Autodesk Inventor part; units mm, degrees
(part 2 of 2)
sketch "Sketch5" plane through (0, 0, 0) normal (0, -1, 0) x (1, 0, 0)
  circle A0 centre (-0.4117, 0.4117) radius 0.057 projected
  line L0 (-0.0797, 0.4378) -> (-0.0785, 0.4393) projected
  line L1 (-0.0785, 0.4393) -> (-0.0772, 0.4404) projected
  line L2 (-0.0772, 0.4404) -> (-0.076, 0.4413) projected
  line L3 (-0.076, 0.4413) -> (-0.0747, 0.442) projected
  line L4 (-0.0747, 0.442) -> (-0.0734, 0.4426) projected
  line L5 (-0.0734, 0.4426) -> (-0.0708, 0.4437) projected
  line L6 (-0.0708, 0.4437) -> (-0.0682, 0.4445) projected
  line L7 (-0.0682, 0.4445) -> (-0.0656, 0.4451) projected
  line L8 (-0.0656, 0.4451) -> (-0.0604, 0.4462) projected
  line L9 (-0.0604, 0.4462) -> (-0.0552, 0.4478) projected
  line L10 (-0.0552, 0.4478) -> (-0.05, 0.4497) projected
  line L11 (-0.05, 0.4497) -> (-0.0449, 0.452) projected
  line L12 (-0.0449, 0.452) -> (-0.0398, 0.4545) projected
  line L13 (-0.0398, 0.4545) -> (-0.0348, 0.4573) projected
  line L14 (-0.0348, 0.4573) -> (-0.0298, 0.4603) projected
  line L15 (-0.0298, 0.4603) -> (-0.0248, 0.4636) projected
  line L16 (-0.0248, 0.4636) -> (-0.0199, 0.467) projected
  line L17 (-0.0199, 0.467) -> (-0.015, 0.4707) projected
  line L18 (-0.015, 0.4707) -> (-0.0102, 0.4745) projected
  line L19 (-0.0102, 0.4745) -> (-0.0055, 0.4786) projected
  line L20 (-0.0055, 0.4786) -> (-0.0167, 0.5276) projected
  line L21 (-0.0167, 0.5276) -> (-0.0227, 0.5292) projected
  line L22 (-0.0227, 0.5292) -> (-0.0287, 0.5306) projected
  line L23 (-0.0287, 0.5306) -> (-0.0347, 0.5318) projected
  line L24 (-0.0347, 0.5318) -> (-0.0406, 0.5328) projected
  line L25 (-0.0406, 0.5328) -> (-0.0465, 0.5335) projected
  line L26 (-0.0465, 0.5335) -> (-0.0523, 0.5341) projected
  line L27 (-0.0523, 0.5341) -> (-0.058, 0.5344) projected
  line L28 (-0.058, 0.5344) -> (-0.0637, 0.5345) projected
  line L29 (-0.0637, 0.5345) -> (-0.0693, 0.5343) projected
  line L30 (-0.0693, 0.5343) -> (-0.0748, 0.5338) projected
  line L31 (-0.0748, 0.5338) -> (-0.0802, 0.5329) projected
  line L32 (-0.0802, 0.5329) -> (-0.0854, 0.5316) projected
  line L33 (-0.0854, 0.5316) -> (-0.088, 0.5311) projected
  line L34 (-0.088, 0.5311) -> (-0.0907, 0.5307) projected
  line L35 (-0.0907, 0.5307) -> (-0.0935, 0.5305) projected
  line L36 (-0.0935, 0.5305) -> (-0.0949, 0.5305) projected
  line L37 (-0.0949, 0.5305) -> (-0.0964, 0.5307) projected
  line L38 (-0.0964, 0.5307) -> (-0.0979, 0.5309) projected
  line L39 (-0.0979, 0.5309) -> (-0.0995, 0.5313) projected
  line L40 (-0.0995, 0.5313) -> (-0.1012, 0.5322) projected
  line L41 (-0.1012, 0.5322) -> (-0.1038, 0.535) projected
  line L42 (-0.1038, 0.535) -> (-0.1233, 0.5755) projected
  line L43 (-0.1233, 0.5755) -> (-0.1239, 0.5792) projected
  line L44 (-0.1239, 0.5792) -> (-0.1235, 0.5811) projected
  line L45 (-0.1235, 0.5811) -> (-0.1228, 0.5826) projected
  line L46 (-0.1228, 0.5826) -> (-0.1221, 0.584) projected
  line L47 (-0.1221, 0.584) -> (-0.1212, 0.5852) projected
  line L48 (-0.1212, 0.5852) -> (-0.1204, 0.5863) projected
  line L49 (-0.1204, 0.5863) -> (-0.1185, 0.5884) projected
  line L50 (-0.1185, 0.5884) -> (-0.1165, 0.5903) projected
  line L51 (-0.1165, 0.5903) -> (-0.1144, 0.592) projected
  line L52 (-0.1144, 0.592) -> (-0.1102, 0.5952) projected
  line L53 (-0.1102, 0.5952) -> (-0.1061, 0.5989) projected
  line L54 (-0.1061, 0.5989) -> (-0.1023, 0.6029) projected
  line L55 (-0.1023, 0.6029) -> (-0.0987, 0.6071) projected
  line L56 (-0.0987, 0.6071) -> (-0.0952, 0.6116) projected
  line L57 (-0.0952, 0.6116) -> (-0.0919, 0.6163) projected
  line L58 (-0.0919, 0.6163) -> (-0.0887, 0.6212) projected
  line L59 (-0.0887, 0.6212) -> (-0.0856, 0.6263) projected
  line L60 (-0.0856, 0.6263) -> (-0.0827, 0.6315) projected
  line L61 (-0.0827, 0.6315) -> (-0.0799, 0.6369) projected
  line L62 (-0.0799, 0.6369) -> (-0.0773, 0.6425) projected
  line L63 (-0.0773, 0.6425) -> (-0.0747, 0.6482) projected
  line L64 (-0.0747, 0.6482) -> (-0.1061, 0.6875) projected
  line L65 (-0.1061, 0.6875) -> (-0.1122, 0.6863) projected
  line L66 (-0.1122, 0.6863) -> (-0.1182, 0.685) projected
  line L67 (-0.1182, 0.685) -> (-0.1241, 0.6835) projected
  line L68 (-0.1241, 0.6835) -> (-0.1299, 0.6818) projected
  line L69 (-0.1299, 0.6818) -> (-0.1355, 0.6799) projected
  line L70 (-0.1355, 0.6799) -> (-0.141, 0.6779) projected
  line L71 (-0.141, 0.6779) -> (-0.1463, 0.6757) projected
  line L72 (-0.1463, 0.6757) -> (-0.1515, 0.6733) projected
  line L73 (-0.1515, 0.6733) -> (-0.1564, 0.6707) projected
  line L74 (-0.1564, 0.6707) -> (-0.1612, 0.6679) projected
  line L75 (-0.1612, 0.6679) -> (-0.1656, 0.6648) projected
  line L76 (-0.1656, 0.6648) -> (-0.1697, 0.6613) projected
  line L77 (-0.1697, 0.6613) -> (-0.1719, 0.6597) projected
  line L78 (-0.1719, 0.6597) -> (-0.1741, 0.6582) projected
  line L79 (-0.1741, 0.6582) -> (-0.1766, 0.6568) projected
  line L80 (-0.1766, 0.6568) -> (-0.1779, 0.6562) projected
  line L81 (-0.1779, 0.6562) -> (-0.1792, 0.6557) projected
  line L82 (-0.1792, 0.6557) -> (-0.1807, 0.6552) projected
  line L83 (-0.1807, 0.6552) -> (-0.1823, 0.6549) projected
  line L84 (-0.1823, 0.6549) -> (-0.1843, 0.6549) projected
  line L85 (-0.1843, 0.6549) -> (-0.1878, 0.6564) projected
  line L86 (-0.1878, 0.6564) -> (-0.2229, 0.6844) projected
  line L87 (-0.2229, 0.6844) -> (-0.2251, 0.6875) projected
  line L88 (-0.2251, 0.6875) -> (-0.2255, 0.6894) projected
  line L89 (-0.2255, 0.6894) -> (-0.2256, 0.691) projected
  line L90 (-0.2256, 0.691) -> (-0.2255, 0.6926) projected
  line L91 (-0.2255, 0.6926) -> (-0.2253, 0.694) projected
  line L92 (-0.2253, 0.694) -> (-0.225, 0.6954) projected
  line L93 (-0.225, 0.6954) -> (-0.2242, 0.6981) projected
  line L94 (-0.2242, 0.6981) -> (-0.2232, 0.7006) projected
  line L95 (-0.2232, 0.7006) -> (-0.2221, 0.7031) projected
  line L96 (-0.2221, 0.7031) -> (-0.2197, 0.7079) projected
  line L97 (-0.2197, 0.7079) -> (-0.2176, 0.7129) projected
  line L98 (-0.2176, 0.7129) -> (-0.2159, 0.7181) projected
  line L99 (-0.2159, 0.7181) -> (-0.2145, 0.7236) projected
  line L100 (-0.2145, 0.7236) -> (-0.2133, 0.7291) projected
  line L101 (-0.2133, 0.7291) -> (-0.2123, 0.7348) projected
  line L102 (-0.2123, 0.7348) -> (-0.2116, 0.7406) projected
  line L103 (-0.2116, 0.7406) -> (-0.211, 0.7465) projected
  line L104 (-0.211, 0.7465) -> (-0.2107, 0.7525) projected
  line L105 (-0.2107, 0.7525) -> (-0.2105, 0.7585) projected
  line L106 (-0.2105, 0.7585) -> (-0.2105, 0.7647) projected
  line L107 (-0.2105, 0.7647) -> (-0.2107, 0.771) projected
  line L108 (-0.2107, 0.771) -> (-0.256, 0.7928) projected
  line L109 (-0.256, 0.7928) -> (-0.261, 0.789) projected
  line L110 (-0.261, 0.789) -> (-0.2659, 0.7852) projected
  line L111 (-0.2659, 0.7852) -> (-0.2705, 0.7813) projected
  line L112 (-0.2705, 0.7813) -> (-0.275, 0.7773) projected
  line L113 (-0.275, 0.7773) -> (-0.2793, 0.7732) projected
  line L114 (-0.2793, 0.7732) -> (-0.2833, 0.769) projected
  line L115 (-0.2833, 0.769) -> (-0.2872, 0.7647) projected
  line L116 (-0.2872, 0.7647) -> (-0.2908, 0.7603) projected
  line L117 (-0.2908, 0.7603) -> (-0.2941, 0.7558) projected
  line L118 (-0.2941, 0.7558) -> (-0.2971, 0.7512) projected
  line L119 (-0.2971, 0.7512) -> (-0.2998, 0.7465) projected
  line L120 (-0.2998, 0.7465) -> (-0.302, 0.7416) projected
  line L121 (-0.302, 0.7416) -> (-0.3032, 0.7392) projected
  line L122 (-0.3032, 0.7392) -> (-0.3046, 0.7368) projected
  line L123 (-0.3046, 0.7368) -> (-0.3062, 0.7345) projected
  line L124 (-0.3062, 0.7345) -> (-0.3071, 0.7334) projected
  line L125 (-0.3071, 0.7334) -> (-0.3081, 0.7323) projected
  line L126 (-0.3081, 0.7323) -> (-0.3093, 0.7313) projected
  line L127 (-0.3093, 0.7313) -> (-0.3106, 0.7303) projected
  line L128 (-0.3106, 0.7303) -> (-0.3123, 0.7295) projected
  line L129 (-0.3123, 0.7295) -> (-0.3161, 0.7293) projected
  line L130 (-0.3161, 0.7293) -> (-0.3599, 0.7393) projected
  line L131 (-0.3599, 0.7393) -> (-0.3633, 0.7411) projected
  line L132 (-0.3633, 0.7411) -> (-0.3644, 0.7426) projected
  line L133 (-0.3644, 0.7426) -> (-0.3652, 0.7441) projected
  line L134 (-0.3652, 0.7441) -> (-0.3658, 0.7455) projected
  line L135 (-0.3658, 0.7455) -> (-0.3663, 0.7469) projected
  line L136 (-0.3663, 0.7469) -> (-0.3666, 0.7483) projected
  line L137 (-0.3666, 0.7483) -> (-0.3671, 0.7511) projected
  line L138 (-0.3671, 0.7511) -> (-0.3673, 0.7538) projected
  line L139 (-0.3673, 0.7538) -> (-0.3673, 0.7565) projected
  line L140 (-0.3673, 0.7565) -> (-0.3672, 0.7618) projected
  line L141 (-0.3672, 0.7618) -> (-0.3676, 0.7673) projected
  line L142 (-0.3676, 0.7673) -> (-0.3683, 0.7727) projected
  line L143 (-0.3683, 0.7727) -> (-0.3694, 0.7782) projected
  line L144 (-0.3694, 0.7782) -> (-0.3707, 0.7837) projected
  line L145 (-0.3707, 0.7837) -> (-0.3723, 0.7893) projected
  line L146 (-0.3723, 0.7893) -> (-0.3741, 0.7948) projected
  line L147 (-0.3741, 0.7948) -> (-0.3762, 0.8004) projected
  line L148 (-0.3762, 0.8004) -> (-0.3784, 0.8059) projected
  line L149 (-0.3784, 0.8059) -> (-0.3809, 0.8115) projected
  line L150 (-0.3809, 0.8115) -> (-0.3836, 0.817) projected
  line L151 (-0.3836, 0.817) -> (-0.3865, 0.8226) projected
  line L152 (-0.3865, 0.8226) -> (-0.4368, 0.8226) projected
  line L153 (-0.4368, 0.8226) -> (-0.4397, 0.817) projected
  line L154 (-0.4397, 0.817) -> (-0.4424, 0.8115) projected
  line L155 (-0.4424, 0.8115) -> (-0.4449, 0.8059) projected
  line L156 (-0.4449, 0.8059) -> (-0.4472, 0.8004) projected
  line L157 (-0.4472, 0.8004) -> (-0.4492, 0.7948) projected
  line L158 (-0.4492, 0.7948) -> (-0.4511, 0.7893) projected
  line L159 (-0.4511, 0.7893) -> (-0.4527, 0.7837) projected
  line L160 (-0.4527, 0.7837) -> (-0.454, 0.7782) projected
  line L161 (-0.454, 0.7782) -> (-0.455, 0.7727) projected
  line L162 (-0.455, 0.7727) -> (-0.4558, 0.7673) projected
  line L163 (-0.4558, 0.7673) -> (-0.4561, 0.7618) projected
  line L164 (-0.4561, 0.7618) -> (-0.456, 0.7565) projected
  line L165 (-0.456, 0.7565) -> (-0.4561, 0.7538) projected
  line L166 (-0.4561, 0.7538) -> (-0.4563, 0.7511) projected
  line L167 (-0.4563, 0.7511) -> (-0.4567, 0.7483) projected
  line L168 (-0.4567, 0.7483) -> (-0.4571, 0.7469) projected
  line L169 (-0.4571, 0.7469) -> (-0.4575, 0.7455) projected
  line L170 (-0.4575, 0.7455) -> (-0.4581, 0.7441) projected
  line L171 (-0.4581, 0.7441) -> (-0.4589, 0.7426) projected
  line L172 (-0.4589, 0.7426) -> (-0.4601, 0.7411) projected
  line L173 (-0.4601, 0.7411) -> (-0.4634, 0.7393) projected
  line L174 (-0.4634, 0.7393) -> (-0.5072, 0.7293) projected
  line L175 (-0.5072, 0.7293) -> (-0.511, 0.7295) projected
  line L176 (-0.511, 0.7295) -> (-0.5127, 0.7303) projected
  line L177 (-0.5127, 0.7303) -> (-0.5141, 0.7313) projected
  line L178 (-0.5141, 0.7313) -> (-0.5152, 0.7323) projected
  line L179 (-0.5152, 0.7323) -> (-0.5162, 0.7334) projected
  line L180 (-0.5162, 0.7334) -> (-0.5171, 0.7345) projected
  line L181 (-0.5171, 0.7345) -> (-0.5187, 0.7368) projected
  line L182 (-0.5187, 0.7368) -> (-0.5201, 0.7392) projected
  line L183 (-0.5201, 0.7392) -> (-0.5213, 0.7416) projected
  line L184 (-0.5213, 0.7416) -> (-0.5235, 0.7465) projected
  line L185 (-0.5235, 0.7465) -> (-0.5262, 0.7512) projected
  line L186 (-0.5262, 0.7512) -> (-0.5293, 0.7558) projected
  line L187 (-0.5293, 0.7558) -> (-0.5326, 0.7603) projected
  line L188 (-0.5326, 0.7603) -> (-0.5362, 0.7647) projected
  line L189 (-0.5362, 0.7647) -> (-0.54, 0.769) projected
  line L190 (-0.54, 0.769) -> (-0.5441, 0.7732) projected
  line L191 (-0.5441, 0.7732) -> (-0.5483, 0.7773) projected
  line L192 (-0.5483, 0.7773) -> (-0.5528, 0.7813) projected
  line L193 (-0.5528, 0.7813) -> (-0.5575, 0.7852) projected
  line L194 (-0.5575, 0.7852) -> (-0.5623, 0.789) projected
  line L195 (-0.5623, 0.789) -> (-0.5673, 0.7928) projected
  line L196 (-0.5673, 0.7928) -> (-0.6126, 0.771) projected
  line L197 (-0.6126, 0.771) -> (-0.6128, 0.7647) projected
  line L198 (-0.6128, 0.7647) -> (-0.6128, 0.7585) projected
  line L199 (-0.6128, 0.7585) -> (-0.6127, 0.7525) projected
  line L200 (-0.6127, 0.7525) -> (-0.6123, 0.7465) projected
  line L201 (-0.6123, 0.7465) -> (-0.6118, 0.7406) projected
  line L202 (-0.6118, 0.7406) -> (-0.611, 0.7348) projected
  line L203 (-0.611, 0.7348) -> (-0.61, 0.7291) projected
  line L204 (-0.61, 0.7291) -> (-0.6088, 0.7236) projected
  line L205 (-0.6088, 0.7236) -> (-0.6074, 0.7181) projected
  line L206 (-0.6074, 0.7181) -> (-0.6057, 0.7129) projected
  line L207 (-0.6057, 0.7129) -> (-0.6037, 0.7079) projected
  line L208 (-0.6037, 0.7079) -> (-0.6013, 0.7031) projected
  line L209 (-0.6013, 0.7031) -> (-0.6001, 0.7006) projected
  line L210 (-0.6001, 0.7006) -> (-0.5991, 0.6981) projected
  line L211 (-0.5991, 0.6981) -> (-0.5983, 0.6954) projected
  line L212 (-0.5983, 0.6954) -> (-0.598, 0.694) projected
  line L213 (-0.598, 0.694) -> (-0.5978, 0.6926) projected
  line L214 (-0.5978, 0.6926) -> (-0.5977, 0.691) projected
  line L215 (-0.5977, 0.691) -> (-0.5978, 0.6894) projected
  line L216 (-0.5978, 0.6894) -> (-0.5982, 0.6875) projected
  line L217 (-0.5982, 0.6875) -> (-0.6004, 0.6844) projected
  line L218 (-0.6004, 0.6844) -> (-0.6356, 0.6564) projected
  line L219 (-0.6356, 0.6564) -> (-0.6391, 0.6549) projected
  line L220 (-0.6391, 0.6549) -> (-0.641, 0.6549) projected
  line L221 (-0.641, 0.6549) -> (-0.6426, 0.6552) projected
  line L222 (-0.6426, 0.6552) -> (-0.6441, 0.6557) projected
  line L223 (-0.6441, 0.6557) -> (-0.6455, 0.6562) projected
  line L224 (-0.6455, 0.6562) -> (-0.6468, 0.6568) projected
  line L225 (-0.6468, 0.6568) -> (-0.6492, 0.6582) projected
  line L226 (-0.6492, 0.6582) -> (-0.6515, 0.6597) projected
  line L227 (-0.6515, 0.6597) -> (-0.6536, 0.6613) projected
  line L228 (-0.6536, 0.6613) -> (-0.6577, 0.6648) projected
  line L229 (-0.6577, 0.6648) -> (-0.6622, 0.6679) projected
  line L230 (-0.6622, 0.6679) -> (-0.6669, 0.6707) projected
  line L231 (-0.6669, 0.6707) -> (-0.6719, 0.6733) projected
  line L232 (-0.6719, 0.6733) -> (-0.677, 0.6757) projected
  line L233 (-0.677, 0.6757) -> (-0.6823, 0.6779) projected
  line L234 (-0.6823, 0.6779) -> (-0.6878, 0.6799) projected
  line L235 (-0.6878, 0.6799) -> (-0.6935, 0.6818) projected
  line L236 (-0.6935, 0.6818) -> (-0.6992, 0.6835) projected
  line L237 (-0.6992, 0.6835) -> (-0.7051, 0.685) projected
  line L238 (-0.7051, 0.685) -> (-0.7111, 0.6863) projected
  line L239 (-0.7111, 0.6863) -> (-0.7173, 0.6875) projected
  line L240 (-0.7173, 0.6875) -> (-0.7486, 0.6482) projected
  line L241 (-0.7486, 0.6482) -> (-0.7461, 0.6425) projected
  line L242 (-0.7461, 0.6425) -> (-0.7434, 0.6369) projected
  line L243 (-0.7434, 0.6369) -> (-0.7406, 0.6315) projected
  line L244 (-0.7406, 0.6315) -> (-0.7377, 0.6263) projected
  line L245 (-0.7377, 0.6263) -> (-0.7347, 0.6212) projected
  line L246 (-0.7347, 0.6212) -> (-0.7315, 0.6163) projected
  line L247 (-0.7315, 0.6163) -> (-0.7281, 0.6116) projected
  line L248 (-0.7281, 0.6116) -> (-0.7247, 0.6071) projected
  line L249 (-0.7247, 0.6071) -> (-0.721, 0.6029) projected
  line L250 (-0.721, 0.6029) -> (-0.7172, 0.5989) projected
  line L251 (-0.7172, 0.5989) -> (-0.7132, 0.5952) projected
  line L252 (-0.7132, 0.5952) -> (-0.7089, 0.592) projected
  line L253 (-0.7089, 0.592) -> (-0.7068, 0.5903) projected
  line L254 (-0.7068, 0.5903) -> (-0.7049, 0.5884) projected
  line L255 (-0.7049, 0.5884) -> (-0.703, 0.5863) projected
  line L256 (-0.703, 0.5863) -> (-0.7021, 0.5852) projected
  line L257 (-0.7021, 0.5852) -> (-0.7013, 0.584) projected
  line L258 (-0.7013, 0.584) -> (-0.7005, 0.5826) projected
  line L259 (-0.7005, 0.5826) -> (-0.6999, 0.5811) projected
  line L260 (-0.6999, 0.5811) -> (-0.6994, 0.5792) projected
  line L261 (-0.6994, 0.5792) -> (-0.7001, 0.5755) projected
  line L262 (-0.7001, 0.5755) -> (-0.7196, 0.535) projected
  line L263 (-0.7196, 0.535) -> (-0.7221, 0.5322) projected
  line L264 (-0.7221, 0.5322) -> (-0.7238, 0.5314) projected
  line L265 (-0.7238, 0.5314) -> (-0.7254, 0.5309) projected
  line L266 (-0.7254, 0.5309) -> (-0.727, 0.5307) projected
  line L267 (-0.727, 0.5307) -> (-0.7284, 0.5305) projected
  line L268 (-0.7284, 0.5305) -> (-0.7299, 0.5305) projected
  line L269 (-0.7299, 0.5305) -> (-0.7326, 0.5307) projected
  line L270 (-0.7326, 0.5307) -> (-0.7353, 0.5311) projected
  line L271 (-0.7353, 0.5311) -> (-0.738, 0.5316) projected
  line L272 (-0.738, 0.5316) -> (-0.7432, 0.5329) projected
  line L273 (-0.7432, 0.5329) -> (-0.7485, 0.5338) projected
  line L274 (-0.7485, 0.5338) -> (-0.754, 0.5343) projected
  line L275 (-0.754, 0.5343) -> (-0.7596, 0.5345) projected
  line L276 (-0.7596, 0.5345) -> (-0.7653, 0.5344) projected
  line L277 (-0.7653, 0.5344) -> (-0.7711, 0.5341) projected
  line L278 (-0.7711, 0.5341) -> (-0.7769, 0.5336) projected
  line L279 (-0.7769, 0.5336) -> (-0.7827, 0.5328) projected
  line L280 (-0.7827, 0.5328) -> (-0.7887, 0.5318) projected
  line L281 (-0.7887, 0.5318) -> (-0.7946, 0.5306) projected
  line L282 (-0.7946, 0.5306) -> (-0.8006, 0.5292) projected
  line L283 (-0.8006, 0.5292) -> (-0.8067, 0.5276) projected
  line L284 (-0.8067, 0.5276) -> (-0.8179, 0.4786) projected
  line L285 (-0.8179, 0.4786) -> (-0.8131, 0.4745) projected
  line L286 (-0.8131, 0.4745) -> (-0.8083, 0.4707) projected
  line L287 (-0.8083, 0.4707) -> (-0.8034, 0.467) projected
  line L288 (-0.8034, 0.467) -> (-0.7985, 0.4635) projected
  line L289 (-0.7985, 0.4635) -> (-0.7935, 0.4603) projected
  line L290 (-0.7935, 0.4603) -> (-0.7885, 0.4573) projected
  line L291 (-0.7885, 0.4573) -> (-0.7835, 0.4545) projected
  line L292 (-0.7835, 0.4545) -> (-0.7784, 0.452) projected
  line L293 (-0.7784, 0.452) -> (-0.7733, 0.4497) projected
  line L294 (-0.7733, 0.4497) -> (-0.7681, 0.4478) projected
  line L295 (-0.7681, 0.4478) -> (-0.7629, 0.4463) projected
  line L296 (-0.7629, 0.4463) -> (-0.7577, 0.4452) projected
  line L297 (-0.7577, 0.4452) -> (-0.7551, 0.4445) projected
  line L298 (-0.7551, 0.4445) -> (-0.7525, 0.4437) projected
  line L299 (-0.7525, 0.4437) -> (-0.7499, 0.4427) projected
  line L300 (-0.7499, 0.4427) -> (-0.7486, 0.442) projected
  line L301 (-0.7486, 0.442) -> (-0.7473, 0.4413) projected
  line L302 (-0.7473, 0.4413) -> (-0.7461, 0.4404) projected
  line L303 (-0.7461, 0.4404) -> (-0.7448, 0.4393) projected
  line L304 (-0.7448, 0.4393) -> (-0.7436, 0.4378) projected
  line L305 (-0.7436, 0.4378) -> (-0.7425, 0.4342) projected
  line L306 (-0.7425, 0.4342) -> (-0.7425, 0.3892) projected
  line L307 (-0.7425, 0.3892) -> (-0.7436, 0.3856) projected
  line L308 (-0.7436, 0.3856) -> (-0.7448, 0.3841) projected
  line L309 (-0.7448, 0.3841) -> (-0.7461, 0.383) projected
  line L310 (-0.7461, 0.383) -> (-0.7473, 0.3821) projected
  line L311 (-0.7473, 0.3821) -> (-0.7486, 0.3813) projected
  line L312 (-0.7486, 0.3813) -> (-0.7499, 0.3807) projected
  line L313 (-0.7499, 0.3807) -> (-0.7525, 0.3797) projected
  line L314 (-0.7525, 0.3797) -> (-0.7551, 0.3788) projected
  line L315 (-0.7551, 0.3788) -> (-0.7577, 0.3782) projected
  line L316 (-0.7577, 0.3782) -> (-0.7629, 0.3771) projected
  line L317 (-0.7629, 0.3771) -> (-0.7681, 0.3756) projected
  line L318 (-0.7681, 0.3756) -> (-0.7733, 0.3736) projected
  line L319 (-0.7733, 0.3736) -> (-0.7784, 0.3714) projected
  line L320 (-0.7784, 0.3714) -> (-0.7835, 0.3688) projected
  line L321 (-0.7835, 0.3688) -> (-0.7885, 0.3661) projected
  line L322 (-0.7885, 0.3661) -> (-0.7935, 0.363) projected
  line L323 (-0.7935, 0.363) -> (-0.7985, 0.3598) projected
  line L324 (-0.7985, 0.3598) -> (-0.8034, 0.3563) projected
  line L325 (-0.8034, 0.3563) -> (-0.8083, 0.3527) projected
  line L326 (-0.8083, 0.3527) -> (-0.8131, 0.3488) projected
  line L327 (-0.8131, 0.3488) -> (-0.8179, 0.3447) projected
  line L328 (-0.8179, 0.3447) -> (-0.8067, 0.2957) projected
  line L329 (-0.8067, 0.2957) -> (-0.8006, 0.2941) projected
  line L330 (-0.8006, 0.2941) -> (-0.7946, 0.2927) projected
  line L331 (-0.7946, 0.2927) -> (-0.7887, 0.2915) projected
  line L332 (-0.7887, 0.2915) -> (-0.7827, 0.2906) projected
  line L333 (-0.7827, 0.2906) -> (-0.7769, 0.2898) projected
  line L334 (-0.7769, 0.2898) -> (-0.7711, 0.2892) projected
  line L335 (-0.7711, 0.2892) -> (-0.7653, 0.2889) projected
  line L336 (-0.7653, 0.2889) -> (-0.7596, 0.2888) projected
  line L337 (-0.7596, 0.2888) -> (-0.754, 0.289) projected
  line L338 (-0.754, 0.289) -> (-0.7485, 0.2895) projected
  line L339 (-0.7485, 0.2895) -> (-0.7432, 0.2904) projected
  line L340 (-0.7432, 0.2904) -> (-0.738, 0.2917) projected
  line L341 (-0.738, 0.2917) -> (-0.7353, 0.2923) projected
  line L342 (-0.7353, 0.2923) -> (-0.7326, 0.2927) projected
  line L343 (-0.7326, 0.2927) -> (-0.7299, 0.2928) projected
  line L344 (-0.7299, 0.2928) -> (-0.7284, 0.2928) projected
  line L345 (-0.7284, 0.2928) -> (-0.727, 0.2927) projected
  line L346 (-0.727, 0.2927) -> (-0.7254, 0.2924) projected
  line L347 (-0.7254, 0.2924) -> (-0.7238, 0.292) projected
  line L348 (-0.7238, 0.292) -> (-0.7221, 0.2912) projected
  line L349 (-0.7221, 0.2912) -> (-0.7196, 0.2883) projected
  line L350 (-0.7196, 0.2883) -> (-0.7001, 0.2479) projected
  line L351 (-0.7001, 0.2479) -> (-0.6994, 0.2441) projected
  line L352 (-0.6994, 0.2441) -> (-0.6999, 0.2422) projected
  line L353 (-0.6999, 0.2422) -> (-0.7005, 0.2407) projected
  line L354 (-0.7005, 0.2407) -> (-0.7013, 0.2394) projected
  line L355 (-0.7013, 0.2394) -> (-0.7021, 0.2381) projected
  line L356 (-0.7021, 0.2381) -> (-0.703, 0.237) projected
  line L357 (-0.703, 0.237) -> (-0.7049, 0.2349) projected
  line L358 (-0.7049, 0.2349) -> (-0.7068, 0.2331) projected
  line L359 (-0.7068, 0.2331) -> (-0.7089, 0.2314) projected
  line L360 (-0.7089, 0.2314) -> (-0.7132, 0.2281) projected
  line L361 (-0.7132, 0.2281) -> (-0.7172, 0.2244) projected
  line L362 (-0.7172, 0.2244) -> (-0.721, 0.2205) projected
  line L363 (-0.721, 0.2205) -> (-0.7247, 0.2162) projected
  line L364 (-0.7247, 0.2162) -> (-0.7281, 0.2117) projected
  line L365 (-0.7281, 0.2117) -> (-0.7315, 0.207) projected
  line L366 (-0.7315, 0.207) -> (-0.7347, 0.2021) projected
  line L367 (-0.7347, 0.2021) -> (-0.7377, 0.1971) projected
  line L368 (-0.7377, 0.1971) -> (-0.7406, 0.1918) projected
  line L369 (-0.7406, 0.1918) -> (-0.7434, 0.1864) projected
  line L370 (-0.7434, 0.1864) -> (-0.7461, 0.1809) projected
  line L371 (-0.7461, 0.1809) -> (-0.7486, 0.1751) projected
  line L372 (-0.7486, 0.1751) -> (-0.7173, 0.1358) projected
  line L373 (-0.7173, 0.1358) -> (-0.7111, 0.137) projected
  line L374 (-0.7111, 0.137) -> (-0.7051, 0.1384) projected
  line L375 (-0.7051, 0.1384) -> (-0.6992, 0.1399) projected
  line L376 (-0.6992, 0.1399) -> (-0.6935, 0.1416) projected
  line L377 (-0.6935, 0.1416) -> (-0.6878, 0.1434) projected
  line L378 (-0.6878, 0.1434) -> (-0.6823, 0.1454) projected
  line L379 (-0.6823, 0.1454) -> (-0.677, 0.1476) projected
  line L380 (-0.677, 0.1476) -> (-0.6719, 0.15) projected
  line L381 (-0.6719, 0.15) -> (-0.6669, 0.1526) projected
  line L382 (-0.6669, 0.1526) -> (-0.6622, 0.1555) projected
  line L383 (-0.6622, 0.1555) -> (-0.6577, 0.1586) projected
  line L384 (-0.6577, 0.1586) -> (-0.6536, 0.162) projected
  line L385 (-0.6536, 0.162) -> (-0.6515, 0.1637) projected
  line L386 (-0.6515, 0.1637) -> (-0.6492, 0.1652) projected
  line L387 (-0.6492, 0.1652) -> (-0.6468, 0.1665) projected
  line L388 (-0.6468, 0.1665) -> (-0.6455, 0.1671) projected
  line L389 (-0.6455, 0.1671) -> (-0.6441, 0.1677) projected
  line L390 (-0.6441, 0.1677) -> (-0.6426, 0.1681) projected
  line L391 (-0.6426, 0.1681) -> (-0.641, 0.1684) projected
  line L392 (-0.641, 0.1684) -> (-0.6391, 0.1684) projected
  line L393 (-0.6391, 0.1684) -> (-0.6356, 0.167) projected
  line L394 (-0.6356, 0.167) -> (-0.6004, 0.139) projected
  line L395 (-0.6004, 0.139) -> (-0.5982, 0.1358) projected
  line L396 (-0.5982, 0.1358) -> (-0.5978, 0.134) projected
  line L397 (-0.5978, 0.134) -> (-0.5977, 0.1323) projected
  line L398 (-0.5977, 0.1323) -> (-0.5978, 0.1308) projected
  line L399 (-0.5978, 0.1308) -> (-0.598, 0.1293) projected
  line L400 (-0.598, 0.1293) -> (-0.5983, 0.1279) projected
  line L401 (-0.5983, 0.1279) -> (-0.5991, 0.1252) projected
  line L402 (-0.5991, 0.1252) -> (-0.6001, 0.1227) projected
  line L403 (-0.6001, 0.1227) -> (-0.6013, 0.1203) projected
  line L404 (-0.6013, 0.1203) -> (-0.6037, 0.1155) projected
  line L405 (-0.6037, 0.1155) -> (-0.6057, 0.1104) projected
  line L406 (-0.6057, 0.1104) -> (-0.6074, 0.1052) projected
  line L407 (-0.6074, 0.1052) -> (-0.6088, 0.0998) projected
  line L408 (-0.6088, 0.0998) -> (-0.61, 0.0942) projected
  line L409 (-0.61, 0.0942) -> (-0.611, 0.0885) projected
  line L410 (-0.611, 0.0885) -> (-0.6118, 0.0828) projected
  line L411 (-0.6118, 0.0828) -> (-0.6123, 0.0769) projected
  line L412 (-0.6123, 0.0769) -> (-0.6127, 0.0709) projected
  line L413 (-0.6127, 0.0709) -> (-0.6128, 0.0648) projected
  line L414 (-0.6128, 0.0648) -> (-0.6128, 0.0586) projected
  line L415 (-0.6128, 0.0586) -> (-0.6126, 0.0524) projected
  line L416 (-0.6126, 0.0524) -> (-0.5673, 0.0306) projected
  line L417 (-0.5673, 0.0306) -> (-0.5623, 0.0343) projected
  line L418 (-0.5623, 0.0343) -> (-0.5575, 0.0381) projected
  line L419 (-0.5575, 0.0381) -> (-0.5528, 0.042) projected
  line L420 (-0.5528, 0.042) -> (-0.5483, 0.046) projected
  line L421 (-0.5483, 0.046) -> (-0.5441, 0.0502) projected
  line L422 (-0.5441, 0.0502) -> (-0.54, 0.0544) projected
  line L423 (-0.54, 0.0544) -> (-0.5362, 0.0587) projected
  line L424 (-0.5362, 0.0587) -> (-0.5326, 0.0631) projected
  line L425 (-0.5326, 0.0631) -> (-0.5293, 0.0675) projected
  line L426 (-0.5293, 0.0675) -> (-0.5262, 0.0721) projected
  line L427 (-0.5262, 0.0721) -> (-0.5235, 0.0769) projected
  line L428 (-0.5235, 0.0769) -> (-0.5213, 0.0818) projected
  line L429 (-0.5213, 0.0818) -> (-0.5201, 0.0842) projected
  line L430 (-0.5201, 0.0842) -> (-0.5187, 0.0865) projected
  line L431 (-0.5187, 0.0865) -> (-0.5171, 0.0888) projected
  line L432 (-0.5171, 0.0888) -> (-0.5162, 0.0899) projected
  line L433 (-0.5162, 0.0899) -> (-0.5152, 0.091) projected
  line L434 (-0.5152, 0.091) -> (-0.5141, 0.092) projected
  line L435 (-0.5141, 0.092) -> (-0.5127, 0.093) projected
  line L436 (-0.5127, 0.093) -> (-0.511, 0.0938) projected
  line L437 (-0.511, 0.0938) -> (-0.5072, 0.0941) projected
  line L438 (-0.5072, 0.0941) -> (-0.4634, 0.0841) projected
  line L439 (-0.4634, 0.0841) -> (-0.4601, 0.0822) projected
  line L440 (-0.4601, 0.0822) -> (-0.4589, 0.0807) projected
  line L441 (-0.4589, 0.0807) -> (-0.4581, 0.0792) projected
  line L442 (-0.4581, 0.0792) -> (-0.4575, 0.0778) projected
  line L443 (-0.4575, 0.0778) -> (-0.4571, 0.0764) projected
  line L444 (-0.4571, 0.0764) -> (-0.4567, 0.075) projected
  line L445 (-0.4567, 0.075) -> (-0.4563, 0.0723) projected
  line L446 (-0.4563, 0.0723) -> (-0.4561, 0.0695) projected
  line L447 (-0.4561, 0.0695) -> (-0.456, 0.0669) projected
  line L448 (-0.456, 0.0669) -> (-0.4561, 0.0615) projected
  line L449 (-0.4561, 0.0615) -> (-0.4558, 0.0561) projected
  line L450 (-0.4558, 0.0561) -> (-0.455, 0.0506) projected
  line L451 (-0.455, 0.0506) -> (-0.454, 0.0451) projected
  line L452 (-0.454, 0.0451) -> (-0.4527, 0.0396) projected
  line L453 (-0.4527, 0.0396) -> (-0.4511, 0.0341) projected
  line L454 (-0.4511, 0.0341) -> (-0.4492, 0.0285) projected
  line L455 (-0.4492, 0.0285) -> (-0.4472, 0.023) projected
  line L456 (-0.4472, 0.023) -> (-0.4449, 0.0174) projected
  line L457 (-0.4449, 0.0174) -> (-0.4424, 0.0119) projected
  line L458 (-0.4424, 0.0119) -> (-0.4397, 0.0063) projected
  line L459 (-0.4397, 0.0063) -> (-0.4368, 0.0008) projected
  line L460 (-0.4368, 0.0008) -> (-0.3865, 0.0008) projected
  line L461 (-0.3865, 0.0008) -> (-0.3836, 0.0063) projected
  line L462 (-0.3836, 0.0063) -> (-0.3809, 0.0119) projected
  line L463 (-0.3809, 0.0119) -> (-0.3784, 0.0174) projected
  line L464 (-0.3784, 0.0174) -> (-0.3762, 0.023) projected
  line L465 (-0.3762, 0.023) -> (-0.3741, 0.0285) projected
  line L466 (-0.3741, 0.0285) -> (-0.3723, 0.0341) projected
  line L467 (-0.3723, 0.0341) -> (-0.3707, 0.0396) projected
  line L468 (-0.3707, 0.0396) -> (-0.3694, 0.0451) projected
  line L469 (-0.3694, 0.0451) -> (-0.3683, 0.0506) projected
  line L470 (-0.3683, 0.0506) -> (-0.3676, 0.0561) projected
  line L471 (-0.3676, 0.0561) -> (-0.3672, 0.0615) projected
  line L472 (-0.3672, 0.0615) -> (-0.3673, 0.0669) projected
  line L473 (-0.3673, 0.0669) -> (-0.3673, 0.0695) projected
  line L474 (-0.3673, 0.0695) -> (-0.3671, 0.0723) projected
  line L475 (-0.3671, 0.0723) -> (-0.3666, 0.075) projected
  line L476 (-0.3666, 0.075) -> (-0.3663, 0.0764) projected
  line L477 (-0.3663, 0.0764) -> (-0.3658, 0.0778) projected
  line L478 (-0.3658, 0.0778) -> (-0.3652, 0.0792) projected
  line L479 (-0.3652, 0.0792) -> (-0.3644, 0.0807) projected
  line L480 (-0.3644, 0.0807) -> (-0.3633, 0.0822) projected
  line L481 (-0.3633, 0.0822) -> (-0.3599, 0.0841) projected
  line L482 (-0.3599, 0.0841) -> (-0.3161, 0.0941) projected
  line L483 (-0.3161, 0.0941) -> (-0.3123, 0.0938) projected
  line L484 (-0.3123, 0.0938) -> (-0.3106, 0.093) projected
  line L485 (-0.3106, 0.093) -> (-0.3093, 0.092) projected
  line L486 (-0.3093, 0.092) -> (-0.3081, 0.091) projected
  line L487 (-0.3081, 0.091) -> (-0.3071, 0.0899) projected
  line L488 (-0.3071, 0.0899) -> (-0.3062, 0.0888) projected
  line L489 (-0.3062, 0.0888) -> (-0.3046, 0.0865) projected
  line L490 (-0.3046, 0.0865) -> (-0.3032, 0.0842) projected
  line L491 (-0.3032, 0.0842) -> (-0.302, 0.0818) projected
  line L492 (-0.302, 0.0818) -> (-0.2998, 0.0769) projected
  line L493 (-0.2998, 0.0769) -> (-0.2971, 0.0721) projected
  line L494 (-0.2971, 0.0721) -> (-0.2941, 0.0675) projected
  line L495 (-0.2941, 0.0675) -> (-0.2908, 0.0631) projected
  line L496 (-0.2908, 0.0631) -> (-0.2872, 0.0587) projected
  line L497 (-0.2872, 0.0587) -> (-0.2833, 0.0544) projected
  line L498 (-0.2833, 0.0544) -> (-0.2793, 0.0502) projected
  line L499 (-0.2793, 0.0502) -> (-0.275, 0.046) projected
  line L500 (-0.275, 0.046) -> (-0.2705, 0.042) projected
  line L501 (-0.2705, 0.042) -> (-0.2659, 0.0381) projected
  line L502 (-0.2659, 0.0381) -> (-0.261, 0.0343) projected
  line L503 (-0.261, 0.0343) -> (-0.256, 0.0306) projected
  line L504 (-0.256, 0.0306) -> (-0.2107, 0.0524) projected
  line L505 (-0.2107, 0.0524) -> (-0.2105, 0.0586) projected
  line L506 (-0.2105, 0.0586) -> (-0.2105, 0.0648) projected
  line L507 (-0.2105, 0.0648) -> (-0.2107, 0.0709) projected
  line L508 (-0.2107, 0.0709) -> (-0.211, 0.0769) projected
  line L509 (-0.211, 0.0769) -> (-0.2116, 0.0828) projected
  line L510 (-0.2116, 0.0828) -> (-0.2123, 0.0885) projected
  line L511 (-0.2123, 0.0885) -> (-0.2133, 0.0942) projected
  line L512 (-0.2133, 0.0942) -> (-0.2145, 0.0998) projected
  line L513 (-0.2145, 0.0998) -> (-0.2159, 0.1052) projected
  line L514 (-0.2159, 0.1052) -> (-0.2176, 0.1104) projected
  line L515 (-0.2176, 0.1104) -> (-0.2197, 0.1155) projected
  line L516 (-0.2197, 0.1155) -> (-0.2221, 0.1203) projected
  line L517 (-0.2221, 0.1203) -> (-0.2232, 0.1227) projected
  line L518 (-0.2232, 0.1227) -> (-0.2242, 0.1252) projected
  line L519 (-0.2242, 0.1252) -> (-0.225, 0.1279) projected
  line L520 (-0.225, 0.1279) -> (-0.2253, 0.1293) projected
  line L521 (-0.2253, 0.1293) -> (-0.2255, 0.1308) projected
  line L522 (-0.2255, 0.1308) -> (-0.2256, 0.1323) projected
  line L523 (-0.2256, 0.1323) -> (-0.2255, 0.134) projected
  line L524 (-0.2255, 0.134) -> (-0.2251, 0.1358) projected
  line L525 (-0.2251, 0.1358) -> (-0.2229, 0.139) projected
  line L526 (-0.2229, 0.139) -> (-0.1878, 0.167) projected
  line L527 (-0.1878, 0.167) -> (-0.1843, 0.1684) projected
  line L528 (-0.1843, 0.1684) -> (-0.1823, 0.1684) projected
  line L529 (-0.1823, 0.1684) -> (-0.1807, 0.1681) projected
  line L530 (-0.1807, 0.1681) -> (-0.1792, 0.1677) projected
  line L531 (-0.1792, 0.1677) -> (-0.1779, 0.1671) projected
  line L532 (-0.1779, 0.1671) -> (-0.1766, 0.1665) projected
  line L533 (-0.1766, 0.1665) -> (-0.1741, 0.1652) projected
  line L534 (-0.1741, 0.1652) -> (-0.1719, 0.1637) projected
  line L535 (-0.1719, 0.1637) -> (-0.1697, 0.162) projected
  line L536 (-0.1697, 0.162) -> (-0.1656, 0.1586) projected
  line L537 (-0.1656, 0.1586) -> (-0.1612, 0.1555) projected
  line L538 (-0.1612, 0.1555) -> (-0.1564, 0.1526) projected
  line L539 (-0.1564, 0.1526) -> (-0.1515, 0.15) projected
  line L540 (-0.1515, 0.15) -> (-0.1463, 0.1476) projected
  line L541 (-0.1463, 0.1476) -> (-0.141, 0.1454) projected
  line L542 (-0.141, 0.1454) -> (-0.1355, 0.1434) projected
  line L543 (-0.1355, 0.1434) -> (-0.1299, 0.1416) projected
  line L544 (-0.1299, 0.1416) -> (-0.1241, 0.1399) projected
  line L545 (-0.1241, 0.1399) -> (-0.1182, 0.1384) projected
  line L546 (-0.1182, 0.1384) -> (-0.1122, 0.137) projected
  line L547 (-0.1122, 0.137) -> (-0.1061, 0.1358) projected
  line L548 (-0.1061, 0.1358) -> (-0.0747, 0.1751) projected
  line L549 (-0.0747, 0.1751) -> (-0.0773, 0.1809) projected
  line L550 (-0.0773, 0.1809) -> (-0.0799, 0.1864) projected
  line L551 (-0.0799, 0.1864) -> (-0.0827, 0.1918) projected
  line L552 (-0.0827, 0.1918) -> (-0.0856, 0.1971) projected
  line L553 (-0.0856, 0.1971) -> (-0.0887, 0.2021) projected
  line L554 (-0.0887, 0.2021) -> (-0.0919, 0.207) projected
  line L555 (-0.0919, 0.207) -> (-0.0952, 0.2117) projected
  line L556 (-0.0952, 0.2117) -> (-0.0987, 0.2162) projected
  line L557 (-0.0987, 0.2162) -> (-0.1023, 0.2205) projected
  line L558 (-0.1023, 0.2205) -> (-0.1061, 0.2244) projected
  line L559 (-0.1061, 0.2244) -> (-0.1102, 0.2281) projected
  line L560 (-0.1102, 0.2281) -> (-0.1144, 0.2314) projected
  line L561 (-0.1144, 0.2314) -> (-0.1165, 0.2331) projected
  line L562 (-0.1165, 0.2331) -> (-0.1185, 0.2349) projected
  line L563 (-0.1185, 0.2349) -> (-0.1204, 0.237) projected
  line L564 (-0.1204, 0.237) -> (-0.1212, 0.2381) projected
  line L565 (-0.1212, 0.2381) -> (-0.1221, 0.2394) projected
  line L566 (-0.1221, 0.2394) -> (-0.1228, 0.2407) projected
  line L567 (-0.1228, 0.2407) -> (-0.1235, 0.2422) projected
  line L568 (-0.1235, 0.2422) -> (-0.1239, 0.2441) projected
  line L569 (-0.1239, 0.2441) -> (-0.1233, 0.2479) projected
  line L570 (-0.1233, 0.2479) -> (-0.1038, 0.2883) projected
  line L571 (-0.1038, 0.2883) -> (-0.1012, 0.2912) projected
  line L572 (-0.1012, 0.2912) -> (-0.0995, 0.292) projected
  line L573 (-0.0995, 0.292) -> (-0.0979, 0.2924) projected
  line L574 (-0.0979, 0.2924) -> (-0.0964, 0.2927) projected
  line L575 (-0.0964, 0.2927) -> (-0.0949, 0.2928) projected
  line L576 (-0.0949, 0.2928) -> (-0.0935, 0.2928) projected
  line L577 (-0.0935, 0.2928) -> (-0.0907, 0.2927) projected
  line L578 (-0.0907, 0.2927) -> (-0.088, 0.2923) projected
  line L579 (-0.088, 0.2923) -> (-0.0854, 0.2917) projected
  line L580 (-0.0854, 0.2917) -> (-0.0802, 0.2904) projected
  line L581 (-0.0802, 0.2904) -> (-0.0748, 0.2895) projected
  line L582 (-0.0748, 0.2895) -> (-0.0693, 0.289) projected
  line L583 (-0.0693, 0.289) -> (-0.0637, 0.2888) projected
  line L584 (-0.0637, 0.2888) -> (-0.058, 0.2889) projected
  line L585 (-0.058, 0.2889) -> (-0.0523, 0.2892) projected
  line L586 (-0.0523, 0.2892) -> (-0.0465, 0.2898) projected
  line L587 (-0.0465, 0.2898) -> (-0.0406, 0.2906) projected
  line L588 (-0.0406, 0.2906) -> (-0.0347, 0.2915) projected
  line L589 (-0.0347, 0.2915) -> (-0.0287, 0.2927) projected
  line L590 (-0.0287, 0.2927) -> (-0.0227, 0.2941) projected
  line L591 (-0.0227, 0.2941) -> (-0.0167, 0.2957) projected
  line L592 (-0.0167, 0.2957) -> (-0.0055, 0.3447) projected
  line L593 (-0.0055, 0.3447) -> (-0.0102, 0.3488) projected
  line L594 (-0.0102, 0.3488) -> (-0.015, 0.3527) projected
  line L595 (-0.015, 0.3527) -> (-0.0199, 0.3563) projected
  line L596 (-0.0199, 0.3563) -> (-0.0248, 0.3598) projected
  line L597 (-0.0248, 0.3598) -> (-0.0298, 0.363) projected
  line L598 (-0.0298, 0.363) -> (-0.0348, 0.366) projected
  line L599 (-0.0348, 0.366) -> (-0.0398, 0.3688) projected
  line L600 (-0.0398, 0.3688) -> (-0.0449, 0.3714) projected
  line L601 (-0.0449, 0.3714) -> (-0.05, 0.3736) projected
  line L602 (-0.05, 0.3736) -> (-0.0552, 0.3755) projected
  line L603 (-0.0552, 0.3755) -> (-0.0604, 0.3771) projected
  line L604 (-0.0604, 0.3771) -> (-0.0656, 0.3782) projected
  line L605 (-0.0656, 0.3782) -> (-0.0682, 0.3788) projected
  line L606 (-0.0682, 0.3788) -> (-0.0708, 0.3796) projected
  line L607 (-0.0708, 0.3796) -> (-0.0734, 0.3807) projected
  line L608 (-0.0734, 0.3807) -> (-0.0747, 0.3813) projected
  line L609 (-0.0747, 0.3813) -> (-0.076, 0.3821) projected
  line L610 (-0.076, 0.3821) -> (-0.0772, 0.383) projected
  line L611 (-0.0772, 0.383) -> (-0.0785, 0.3841) projected
  line L612 (-0.0785, 0.3841) -> (-0.0797, 0.3855) projected
  line L613 (-0.0797, 0.3855) -> (-0.0808, 0.3892) projected
  line L614 (-0.0808, 0.3892) -> (-0.0808, 0.4341) projected
  line L615 (-0.0808, 0.4341) -> (-0.0797, 0.4378) projected
  point P0 (0, 0)
body "Solid3"
